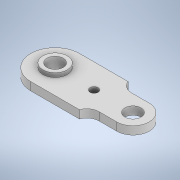
# Autodesk Inventor part: SwivelBase
Saved by Autodesk Inventor 2022.2 (Build 262287030, 287C)
## iProperties
Created: 2023-03-24
Part Number: SwivelBase
Material: Generic
Document SubType Name: Modeling
Designer: jak27277
Density: 1 g/cm^3
Appearance: Default
Author: jak27277
Autodesk Inventor part; units mm, degrees
ref_plane "YZ Plane" through (0, 0, 0) normal (1, 0, 0) x (0, 1, 0)
ref_plane "XZ Plane" through (0, 0, 0) normal (0, 1, 0) x (-1, 0, 0)
ref_plane "XY Plane" through (0, 0, 0) normal (0, 0, 1) x (1, 0, 0)
sketch "Sketch1" plane through (0, 0, 0) normal (0, 1, 0) x (-1, 0, 0)
  arc A0 (0, -30) -> (0, 30) centre (0, 0) ccw
  line L0 (0, -30) -> (-60, -30)
  arc A1 (-60, -30) -> (-74.1421, -20) centre (-74.1421, -35) ccw
  line L1 (-74.1421, -20) -> (-96, -20)
  line L2 (0, 0) -> (-48, 0)
  line L3 (-48, 0) -> (-96, 0)
  line L4 (0, 30) -> (-60, 30)
  arc A2 (-74.1421, 20) -> (-60, 30) centre (-74.1421, 35) ccw
  line L5 (-74.1421, 20) -> (-96, 20)
  arc A3 (-96, 20) -> (-96, -20) centre (-96, 0) ccw
  dimension "d1" = 30
  dimension "d2" = 48
  dimension "d3" = 60
  dimension "d4" = 15
  dimension "d5" = 20
  dimension "d6" = 96
  constraints: 12 end point, 8 point on circle, 5 coincident, 4 centre point, 4 horizontal, 4 symmetric about line, 4 tangent, 1 other
  measures "d1" radius of A0
  measures "d2" distance of L2.start L2.end
  measures "d3" distance of L4.start L4.end
  measures "d4" radius of A1
  measures "d5" radius of A3
  measures "d6" distance of point (-96, 0) point (0, 0)
extrude "Extrusion1" add sketch "Sketch1" along normal blind 10
hole "Hole2" at (0, 0, 0) at (96, 0, 0) direction (0, 1, 0) diameter 20 end through all
hole "Hole3" at (48, 0, 0) at (0, 0, 0) direction (0, 1, 0) diameter 10 end through all
sketch "Sketch3" plane through (0, 10, 0) normal (0, 1, 0) x (1, 0, 0)
  circle A0 centre (0, 0) radius 15
  dimension "d30" = 30
  constraints: 1 centre point, 1 coincident
  measures "d30" diameter of A0
emboss "Emboss1" sketch "Sketch3" operation add depth 5 direction (0, -1, 0)
body "Solid1"
